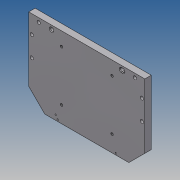
# Autodesk Inventor part: J008086
Saved by Autodesk Inventor 2018.3 (Build 223284000, 284)
## iProperties
Created: 2019-09-03
Material: ALUMINUM, 6061-T651
Vendor: HHMI: JRC - ID&F
Document SubType Name: Modeling
Designer: arnoldj
Density: 2.7 g/cm^3
Appearance: Metal-AL-6061 (Machined)
Part Number: J008086
Description: BBP G STAGE MTG PLATE
Project: COMMON
RuleStatus: InUse
AfterDocSave0: file://Part Number Cleaner
LAB/DEPT: PACHITARIU (LAB)
REQUESTING SCIENTIST: PACHITARIU, MARIUS
SURFACE ROUGHNESS: 63 Ra
DESIGN DEPARTMENT: HHMI: JRC - ID&F
SPECIAL FINISH: ANODIZE PER MIL-A-8625F, TYPE II, CLASS 2 (BLACK)
ALTERED ITEM PART NUMBER: N/A
ALTERED ITEM VENDOR: N/A
ALTERED ITEM DESCRIPTION: N/A
Author: arnoldj
Revision Number: -
Autodesk Inventor part; units mm, degrees
ref_plane "YZ Plane" through (0, 0, 0) normal (1, 0, 0) x (0, 1, 0)
ref_plane "XZ Plane" through (0, 0, 0) normal (0, 1, 0) x (-1, 0, 0)
ref_plane "XY Plane" through (0, 0, 0) normal (0, 0, 1) x (1, 0, 0)
sketch "Sketch1" plane through (0, 0, 0) normal (0, 0, 1) x (1, 0, 0)
  line L0 (0, 111.252) -> (0, -111.887) projected
  line L1 (-161, 0) -> (161, 0) projected
  line L2 (115, -80.01) -> (-115, -80.01)
  line L3 (-115, -80.01) -> (-115, 79.375)
  line L4 (-115, 79.375) -> (115, 79.375)
  line L5 (115, 79.375) -> (115, -80.01)
  line L6 (50, -47.7648) -> (-50, -47.7648) construction
  line L7 (-50, -47.7648) -> (-50, 52.2352) construction
  line L8 (-50, 52.2352) -> (50, 52.2352) construction
  line L9 (50, 52.2352) -> (50, -47.7648) construction
  line L10 (50, -47.7648) -> (-50, 52.2352) construction
  line L11 (-50, -47.7648) -> (50, 52.2352) construction
  line L12 (109, 3.5) -> (-109, 3.5) construction
  line L13 (-109, 3.5) -> (-109, 43.5) construction
  line L14 (-109, 43.5) -> (109, 43.5) construction
  line L15 (109, 43.5) -> (109, 3.5) construction
  line L16 (109, 3.5) -> (-109, 43.5) construction
  line L17 (-109, 3.5) -> (109, 43.5) construction
  point P0 (0, 2.2352)
  point P1 (0, 23.5)
  point P2 (-57.62, -76.7648)
  point P3 (57.62, -76.7648)
  dimension "d0" = 230
  dimension "d1" = 159.385
  dimension "d4" = 100
  dimension "d5" = 100
  dimension "d28" = 35.875
  dimension "d29" = 40
  dimension "d30" = 6
  dimension "d38" = 29
  dimension "d39" = 79.375
  dimension "d40" = 115
  dimension "d48" = 2.2352
  dimension "d52" = 7.62
  dimension "d53" = 7.62
  constraints: 32 end point, 8 coincident, 6 parallel, 4 midpoint, 3 horizontal, 3 perpendicular, 2 point on line, 1 horizontal alignment, 1 other
  measures "d0" distance of L3.end L4.end
  measures "d1" distance of L2.end L3.end
  measures "d4" distance of L7.end L8.end
  measures "d5" distance of L6.end L7.end
  measures "d28" distance between parallel lines of L14 L4
  measures "d29" distance of L12.end L13.end
  measures "d30" distance between parallel lines of L3 L13
  measures "d38" distance from line of L6 point (-57.62, -76.765)
  measures "d39" distance of the line from the sketch origin of L4
  measures "d40" distance between parallel lines of L0 L3
  measures "d52" horizontal distance of point (-50, -47.765) point (-57.62, -76.765)
  measures "d53" horizontal distance of point (50, -47.765) point (57.62, -76.765)
extrude "Extrusion1" add sketch "Sketch1" against normal blind 12.7
hole "Hole1" at (-50, 52.2352, 0) at (50, 52.2352, 0) at (50, -47.7648, 0) at (-50, -47.7648, 0) direction (0, 0, -1) diameter 4.9276 end through all
hole "Hole3" at (-109, 43.5, 0) at (-109, 3.5, 0) at (109, 3.5, 0) at (109, 43.5, 0) direction (0, 0, -1) diameter 6.604 end through all clearance for "Socket Head Cap Screw" size "M6" standard "Ansi Metric M Profile"
chamfer "Chamfer1" distance 31.75 angle 45 2 edges at (-115, -80.01, -6.35) (115, -80.01, -6.35)
sketch "Sketch3" plane through (0, 0, -12.7) normal (0, 0, 1) x (1, 0, 0)
  line L0 (-95.25, 71.4375) -> (95.25, 71.4375) construction
  line L1 (0, 111.252) -> (0, -111.887) construction
  line L2 (-161, 0) -> (161, 0) construction
  line L3 (71.12, 71.4375) -> (68.58, 71.4375) construction
  line L4 (71.12, 74.6252) -> (68.58, 74.6252)
  line L5 (68.58, 68.2498) -> (71.12, 68.2498)
  arc A0 (71.12, 68.2498) -> (71.12, 74.6252) centre (71.12, 71.4375) ccw
  arc A1 (68.58, 74.6252) -> (68.58, 68.2498) centre (68.58, 71.4375) ccw
  line L6 (-115, 79.375) -> (115, 79.375) projected
  point P0 (0, 0)
  point P1 (-69.85, 71.4375)
  point P2 (69.85, 71.4375)
  dimension "d54" = 95.25
  dimension "d55" = 69.85
  dimension "d56" = 69.85
  dimension "d57" = 95.25
  dimension "d58" = 2.54
  dimension "d59" = 6.3754
  dimension "d69" = 7.9375
  constraints: 10 end point, 4 point on circle, 4 tangent, 3 point on line, 2 centre point, 2 coincident, 1 horizontal, 1 midpoint, 1 parallel
  measures "d54" distance from line of L1 point (-95.25, 71.438)
  measures "d55" distance from line of L1 point (-69.85, 71.438)
  measures "d56" distance from line of point (69.85, 71.438) L1
  measures "d57" distance from line of L0.end L1
  measures "d58" distance of L4.start L4.end
  measures "d59" distance between parallel lines of L5 L4
  measures "d69" distance between parallel lines of L0 L6
extrude "Extrusion3" cut sketch "Sketch3" along normal up to next
hole "Hole7" at (-69.85, 71.4375, -12.7) direction (0, 0, 1) diameter 6.3754 end through all
hole "Hole8" at (95.25, 71.4375, -12.7) at (-95.25, 71.4375, -12.7) direction (0, 0, 1) diameter 6.604 end through all clearance for "Socket Head Cap Screw" size "M6" standard "Ansi Metric M Profile"
chamfer "Chamfer3" distance 1.27 angle 45 5 edges at (-69.85, 68.2498, 0) (65.3923, 71.4375, 0) (69.85, 74.6252, 0) (74.3077, 71.4375, 0) (69.85, 68.2498, 0)
sketch "Sketch4" plane through (0, 0, -12.7) normal (0, 0, -1) x (-1, 0, 0)
  line L0 (0, -111.887) -> (0, 111.252) projected
  line L1 (-161, 0) -> (161, 0) projected
  line L2 (60, -77.854) -> (-60, -77.854) construction
  line L3 (-60, -77.854) -> (-60, 77.854) construction
  line L4 (-60, 77.854) -> (60, 77.854) construction
  line L5 (60, 77.854) -> (60, -77.854) construction
  line L6 (60, -77.854) -> (-60, 77.854) construction
  line L7 (-60, -77.854) -> (60, 77.854) construction
  circle A0 centre (61.5, -70.4148) radius 1.5 construction
  point P0 (0, 0)
  point P1 (-57.62, -76.7648)
  point P2 (57.62, -76.7648)
  dimension "d106" = 120
  dimension "d107" = 3
  dimension "d108" = 6.35
  constraints: 12 end point, 2 midpoint, 2 parallel, 1 centre point, 1 coincident, 1 horizontal, 1 perpendicular, 1 tangent
  measures "d106" distance of L3.end L4.end
  measures "d107" diameter of A0
  measures "d108" vertical distance of A0.centre point (57.62, -76.765)
hole "Hole9" at (57.62, -76.7648, -12.7) at (-57.62, -76.7648, -12.7) at (-61.5, -70.4148, -12.7) direction (0, 0, 1) diameter 2.9972 end through all counterbore diameter 3.0226 counterbore depth 1.905
equation "\"d40\" = 0.5 * d0"
equation "\"d56\" = d55"
equation "\"d57\" = d54"
body "Solid1"
